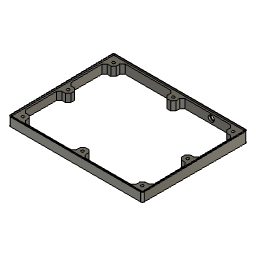
case (Autodesk Fusion 360 design; units mm, degrees)
Autodesk Fusion 360 part; units mm, degrees
sketch "Sketch1" plane through (0, 0, 0) normal (0, 0, 1) x (1, 0, 0)
  line L0 (0, 0) -> (294.692, 0)
  line L1 (294.692, 0) -> (294.692, 230.4)
  line L2 (294.692, 230.4) -> (0, 230.4)
  line L3 (0, 230.4) -> (0, 0)
  line L4 (-2, 232.4) -> (296.692, 232.4)
  line L5 (296.692, 232.4) -> (296.692, -2)
  line L6 (296.692, -2) -> (-2, -2)
  line L7 (-2, -2) -> (-2, 232.4)
  line L8 (4, 226.4) -> (290.692, 226.4)
  line L9 (290.692, 226.4) -> (290.692, 4)
  line L10 (290.692, 4) -> (4, 4)
  line L11 (4, 4) -> (4, 226.4)
  line L12 (4, 226.4) -> (24, 226.4)
  line L13 (24, 226.4) -> (24, 206.4)
  line L14 (24, 206.4) -> (4, 206.4)
  line L15 (4, 206.4) -> (4, 226.4)
  line L16 (-2, 232.4) -> (296.692, -2) construction
  line L17 (-2, -2) -> (296.692, 232.4) construction
  line L18 (-2, 115.2) -> (296.692, 115.2) construction
  line L19 (147.346, 232.4) -> (147.346, -2) construction
  line L20 (4, 206.4) -> (24, 226.4) construction
  line L21 (24, 206.4) -> (4, 226.4) construction
  line L22 (137.346, 226.4) -> (157.346, 226.4)
  line L23 (157.346, 226.4) -> (157.346, 206.4)
  line L24 (157.346, 206.4) -> (137.346, 206.4)
  line L25 (137.346, 206.4) -> (137.346, 226.4)
  line L26 (290.692, 226.4) -> (270.692, 226.4)
  line L27 (270.692, 226.4) -> (270.692, 206.4)
  line L28 (270.692, 206.4) -> (290.692, 206.4)
  line L29 (290.692, 206.4) -> (290.692, 226.4)
  line L30 (4, 125.2) -> (24, 125.2)
  line L31 (24, 125.2) -> (24, 105.2)
  line L32 (24, 105.2) -> (4, 105.2)
  line L33 (4, 105.2) -> (4, 125.2)
  line L34 (290.692, 125.2) -> (270.692, 125.2)
  line L35 (270.692, 125.2) -> (270.692, 105.2)
  line L36 (270.692, 105.2) -> (290.692, 105.2)
  line L37 (290.692, 105.2) -> (290.692, 125.2)
  line L38 (4, 4) -> (24, 4)
  line L39 (24, 4) -> (24, 24)
  line L40 (24, 24) -> (4, 24)
  line L41 (4, 24) -> (4, 4)
  line L42 (137.346, 4) -> (157.346, 4)
  line L43 (157.346, 4) -> (157.346, 24)
  line L44 (157.346, 24) -> (137.346, 24)
  line L45 (137.346, 24) -> (137.346, 4)
  line L46 (290.692, 4) -> (270.692, 4)
  line L47 (270.692, 4) -> (270.692, 24)
  line L48 (270.692, 24) -> (290.692, 24)
  line L49 (290.692, 24) -> (290.692, 4)
  line L50 (137.346, 206.4) -> (157.346, 226.4) construction
  line L51 (157.346, 206.4) -> (137.346, 226.4) construction
  line L52 (270.692, 206.4) -> (290.692, 226.4) construction
  line L53 (290.692, 206.4) -> (270.692, 226.4) construction
  line L54 (270.692, 105.2) -> (290.692, 125.2) construction
  line L55 (290.692, 105.2) -> (270.692, 125.2) construction
  line L56 (4, 105.2) -> (24, 125.2) construction
  line L57 (24, 105.2) -> (4, 125.2) construction
  line L58 (4, 4) -> (24, 24) construction
  line L59 (24, 4) -> (4, 24) construction
  line L60 (137.346, 4) -> (157.346, 24) construction
  line L61 (157.346, 4) -> (137.346, 24) construction
  line L62 (270.692, 4) -> (290.692, 24) construction
  line L63 (290.692, 4) -> (270.692, 24) construction
  circle A0 centre (14, 216.4) radius 3
  circle A1 centre (147.346, 216.4) radius 3
  circle A2 centre (280.692, 216.4) radius 3
  circle A3 centre (14, 115.2) radius 3
  circle A4 centre (280.692, 115.2) radius 3
  circle A5 centre (14, 14) radius 3
  circle A6 centre (147.346, 14) radius 3
  circle A7 centre (280.692, 14) radius 3
  dimension "d1" = 294.692
  dimension "d2" = 230.4
  dimension "d3" = 2
  dimension "d4" = 2
  dimension "d5" = 2
  dimension "d6" = 2
  dimension "d7" = 4
  dimension "d8" = 4
  dimension "d9" = 4
  dimension "d10" = 4
  dimension "d11" = 20
  dimension "d12" = 20
  dimension "d13" = 20
  dimension "d14" = 20
  dimension "d15" = 20
  dimension "d16" = 20
  dimension "d17" = 20
  dimension "d18" = 20
  dimension "d19" = 20
  dimension "d20" = 20
  dimension "d21" = 20
  dimension "d22" = 20
  dimension "d23" = 20
  dimension "d24" = 20
  dimension "d25" = 20
  dimension "d26" = 20
  dimension "d27" = 6
  dimension "d28" = 6
  dimension "d29" = 6
  dimension "d30" = 6
  dimension "d31" = 6
  dimension "d32" = 6
  dimension "d33" = 6
  dimension "d34" = 6
  constraint horizontal L0
  constraint vertical L1
  constraint horizontal L2
  constraint vertical L3
  constraint coincident L0.start L3.end
  constraint horizontal L4
  constraint vertical L5
  constraint horizontal L6
  constraint vertical L7
  constraint horizontal L8
  constraint vertical L9
  constraint horizontal L10
  constraint vertical L11
  constraint horizontal L12
  constraint vertical L13
  constraint horizontal L14
  constraint vertical L15
  constraint midpoint L7 L18.start
  constraint midpoint L5 L18.end
  constraint midpoint L4 L19.start
  constraint midpoint L6 L19.end
  constraint horizontal L22
  constraint vertical L23
  constraint horizontal L24
  constraint vertical L25
  constraint coincident L8 L22.start
  constraint horizontal L26
  constraint vertical L27
  constraint horizontal L28
  constraint vertical L29
  constraint horizontal L30
  constraint vertical L31
  constraint horizontal L32
  constraint vertical L33
  constraint coincident L11 L30.start
  constraint horizontal L34
  constraint vertical L35
  constraint horizontal L36
  constraint vertical L37
  constraint coincident L9 L34.start
  constraint horizontal L38
  constraint vertical L39
  constraint horizontal L40
  constraint vertical L41
  constraint horizontal L42
  constraint vertical L43
  constraint horizontal L44
  constraint vertical L45
  constraint coincident L10 L42.start
  constraint horizontal L46
  constraint vertical L47
  constraint horizontal L48
  constraint vertical L49
  constraint symmetric L19 L23 L25
  constraint symmetric L18 L30 L32
  constraint symmetric L18 L34 L36
  constraint symmetric L19 L43 L45
  constraint midpoint L21 A0.centre
  constraint midpoint L50 A1.centre
  constraint midpoint L53 A2.centre
  constraint midpoint L57 A3.centre
  constraint midpoint L54 A4.centre
  constraint midpoint L59 A5.centre
  constraint midpoint L60 A6.centre
  constraint midpoint L63 A7.centre
  measures "d1" distance of L0.start L0.end
  measures "d2" distance of L0.start L2.end
  measures "d3" distance of L2 L4
  measures "d4" distance of L3 L7
  measures "d5" distance of L0 L6
  measures "d6" distance of L1 L5
  measures "d7" distance of L3 L11
  measures "d8" distance of L0 L10
  measures "d9" distance of L2 L8
  measures "d10" distance of L1 L9
  measures "d11" distance of L8.start L12.end
  measures "d12" distance of L8.start L14.end
  measures "d13" distance of L22.start L22.end
  measures "d14" distance of L22.start L24.end
  measures "d15" distance of L8.end L26.end
  measures "d16" distance of L8.end L28.end
  measures "d17" distance of L30.start L30.end
  measures "d18" distance of L30.start L32.end
  measures "d19" distance of L34.start L34.end
  measures "d20" distance of L34.start L36.end
  measures "d21" distance of L10.end L38.end
  measures "d22" distance of L10.end L40.end
  measures "d23" distance of L42.start L42.end
  measures "d24" distance of L42.start L44.end
  measures "d25" distance of L9.end L46.end
  measures "d26" distance of L9.end L48.end
  measures "d27" diameter of A0
  measures "d28" diameter of A1
  measures "d29" diameter of A2
  measures "d30" diameter of A3
  measures "d31" diameter of A4
  measures "d32" diameter of A5
  measures "d33" diameter of A6
  measures "d34" diameter of A7
extrude "Extrude1" add sketch "Sketch1" along normal blind 20 contours L0 L1 L2 L3 | L4 L5 L6 L7 | L8 L11 L12 L13 L14 L15 | L8 L22 L23 L24 L25 | L11 L30 L31 L32 L33 | L8 L9 L26 L27 L28 L29 | L10 L11 L38 L39 L40 L41 | L9 L34 L35 L36 L37 | L10 L42 L43 L44 L45 | L9 L10 L46 L47 L48 L49
chamfer "Chamfer1" distance 6 angle 45 28 edges at (24, 206.4, 10) (4, 206.4, 10) (24, 226.4, 10) (137.346, 226.4, 10) (137.346, 206.4, 10) (157.346, 206.4, 10) (157.346, 226.4, 10) (270.692, 226.4, 10) (270.692, 206.4, 10) (290.692, 206.4, 10) (290.692, 125.2, 10) (270.692, 125.2, 10) (270.692, 105.2, 10) (290.692, 105.2, 10) (290.692, 24, 10) (270.692, 24, 10) (270.692, 4, 10) (157.346, 4, 10) (157.346, 24, 10) (137.346, 24, 10) (137.346, 4, 10) (24, 4, 10) (24, 24, 10) (4, 24, 10) (24, 105.2, 10) (4, 105.2, 10) (24, 125.2, 10) (4, 125.2, 10)
sketch "Sketch2" plane through (0, 0, 20) normal (0, 0, 1) x (-1, 0, 0)
  line L0 (-24, -119.2) -> (-18, -125.2)
  line L1 (-18, -125.2) -> (-10, -125.2)
  line L2 (-10, -125.2) -> (-4, -131.2)
  line L3 (-4, -131.2) -> (-4, -200.4)
  line L4 (-4, -200.4) -> (-10, -206.4)
  line L5 (-10, -206.4) -> (-18, -206.4)
  line L6 (-18, -206.4) -> (-24, -212.4)
  line L7 (-24, -212.4) -> (-24, -220.4)
  line L8 (-24, -220.4) -> (-30, -226.4)
  line L9 (-30, -226.4) -> (-131.346, -226.4)
  line L10 (-131.346, -226.4) -> (-137.346, -220.4)
  line L11 (-137.346, -220.4) -> (-137.346, -212.4)
  line L12 (-137.346, -212.4) -> (-143.346, -206.4)
  line L13 (-143.346, -206.4) -> (-151.346, -206.4)
  line L14 (-151.346, -206.4) -> (-157.346, -212.4)
  line L15 (-157.346, -212.4) -> (-157.346, -220.4)
  line L16 (-157.346, -220.4) -> (-163.346, -226.4)
  line L17 (-163.346, -226.4) -> (-264.692, -226.4)
  line L18 (-264.692, -226.4) -> (-270.692, -220.4)
  line L19 (-270.692, -220.4) -> (-270.692, -212.4)
  line L20 (-270.692, -212.4) -> (-276.692, -206.4)
  line L21 (-276.692, -206.4) -> (-284.692, -206.4)
  line L22 (-284.692, -206.4) -> (-290.692, -200.4)
  line L23 (-290.692, -200.4) -> (-290.692, -131.2)
  line L24 (-290.692, -131.2) -> (-284.692, -125.2)
  line L25 (-284.692, -125.2) -> (-276.692, -125.2)
  line L26 (-276.692, -125.2) -> (-270.692, -119.2)
  line L27 (-270.692, -119.2) -> (-270.692, -111.2)
  line L28 (-270.692, -111.2) -> (-276.692, -105.2)
  line L29 (-276.692, -105.2) -> (-284.692, -105.2)
  line L30 (-284.692, -105.2) -> (-290.692, -99.2)
  line L31 (-290.692, -99.2) -> (-290.692, -30)
  line L32 (-290.692, -30) -> (-284.692, -24)
  line L33 (-284.692, -24) -> (-276.692, -24)
  line L34 (-276.692, -24) -> (-270.692, -18)
  line L35 (-270.692, -18) -> (-270.692, -10)
  line L36 (-270.692, -10) -> (-264.692, -4)
  line L37 (-264.692, -4) -> (-163.346, -4)
  line L38 (-163.346, -4) -> (-157.346, -10)
  line L39 (-157.346, -10) -> (-157.346, -18)
  line L40 (-157.346, -18) -> (-151.346, -24)
  line L41 (-151.346, -24) -> (-143.346, -24)
  line L42 (-143.346, -24) -> (-137.346, -18)
  line L43 (-137.346, -18) -> (-137.346, -10)
  line L44 (-137.346, -10) -> (-131.346, -4)
  line L45 (-131.346, -4) -> (-30, -4)
  line L46 (-30, -4) -> (-24, -10)
  line L47 (-24, -10) -> (-24, -18)
  line L48 (-24, -18) -> (-18, -24)
  line L49 (-18, -24) -> (-10, -24)
  line L50 (-10, -24) -> (-4, -30)
  line L51 (-4, -30) -> (-4, -99.2)
  line L52 (-4, -99.2) -> (-10, -105.2)
  line L53 (-10, -105.2) -> (-18, -105.2)
  line L54 (-18, -105.2) -> (-24, -111.2)
  line L55 (-24, -111.2) -> (-24, -119.2)
  circle A0 centre (-280.692, -115.2) radius 3
  circle A1 centre (-280.692, -14) radius 3
  circle A2 centre (-147.346, -216.4) radius 3
  circle A3 centre (-14, -115.2) radius 3
  circle A4 centre (-14, -14) radius 3
  circle A5 centre (-280.692, -216.4) radius 3
  circle A6 centre (-147.346, -14) radius 3
  circle A7 centre (-14, -216.4) radius 3
  line L56 (2, 2) -> (-296.692, 2)
  line L57 (-296.692, 2) -> (-296.692, -232.4)
  line L58 (-296.692, -232.4) -> (2, -232.4)
  line L59 (2, -232.4) -> (2, 2)
  line L60 (0, -230.4) -> (-294.692, -230.4)
  line L61 (-294.692, -230.4) -> (-294.692, 0)
  line L62 (-294.692, 0) -> (0, 0)
  line L63 (0, 0) -> (0, -230.4)
  dimension "d38" = 2
  dimension "d39" = 2
  dimension "d40" = 2
  dimension "d41" = 2
  constraint horizontal L60
  constraint vertical L61
  constraint horizontal L62
  constraint vertical L63
  measures "d38" distance of L59 L63
  measures "d39" distance of L58 L60
  measures "d40" distance of L57 L61
  measures "d41" distance of L56 L62
sketch "Sketch3" plane through (-2, 0, 0) normal (-1, 0, 0) x (0, -1, 0)
  line L0 (-232.4, 0) -> (2, 0)
  line L1 (2, 0) -> (2, 20)
  line L2 (2, 20) -> (-232.4, 20)
  line L3 (-232.4, 20) -> (-232.4, 0)
  line L4 (2, 0) -> (2, 16)
  line L5 (2, 16) -> (-232.4, 20)
  dimension "d42" = 16
  constraint coincident L0.end L1.start
  constraint coincident L1 L4.end
  constraint coincident L2.end L3.start
  measures "d42" distance of L0.end L4.end
extrude "Extrude2" cut sketch "Sketch3" against normal through all contours L1 L2 L5
extrude "Extrude3" add sketch "Sketch2" against normal through all of body 1 contours L56 L57 L58 L59
extrude "Extrude4" add 1 faces at (196.4613, -1.3333, 20) along direction (0, 0, 1) blind 3
extrude "Extrude5" add sketch "Sketch1" against normal blind 2 contours L4 L5 L6 L7
sketch "Sketch4" plane through (-2, 0, 0) normal (-1, 0, 0) x (0, -1, 0)
  line L0 (-232.4, 23) -> (-232.4, -2)
  line L1 (-232.4, -2) -> (2, -2)
  line L2 (2, -2) -> (2, 23)
  line L3 (2, 23) -> (-232.4, 23)
  line L4 (2, -2) -> (2, 19)
  line L5 (2, 19) -> (-232.4, 23)
  dimension "d49" = 21
  constraint coincident L1.end L2.start
  constraint perpendicular L3 L4
  constraint coincident L0.start L3.end
  measures "d49" distance of L1.end L4.end
extrude "Extrude6" cut sketch "Sketch4" against normal through all contours L2 L3 L5
sketch "Sketch5" plane through (0, 232.4, 0) normal (0, 1, 0) x (-1, 0, 0)
  line L0 (2, -2) -> (2, 23)
  line L1 (2, 23) -> (-296.692, 23)
  line L2 (-296.692, 23) -> (-296.692, -2)
  line L3 (-296.692, -2) -> (2, -2)
  line L4 (-296.692, -2) -> (2, 23) construction
  line L5 (2, -2) -> (-296.692, 23) construction
  line L6 (-147.346, 23) -> (-147.346, -2) construction
  line L7 (-296.692, -2) -> (-147.346, 23) construction
  line L8 (-147.346, -2) -> (-296.692, 23) construction
  circle A0 centre (-222.019, 10.5) radius 6.3
  circle A1 centre (-222.019, 10.5) radius 6.8
  dimension "d51" = 12.6
  dimension "d52" = 13.6
  constraint coincident L2.end L3.start
  constraint coincident L0.end L1.start
  constraint coincident L0.start L3.end
  constraint coincident L1.end L2.start
  constraint midpoint L1 L6.start
  constraint midpoint L3 L6.end
  constraint midpoint L8 A0.centre
  constraint concentric A0 A1
  measures "d51" diameter of A0
  measures "d52" diameter of A1
extrude "Extrude7" cut sketch "Sketch5" against normal blind 6 contours A0 | A1
extrude "Extrude8" add sketch "Sketch5" against normal blind 2 contours A1
fillet "Fillet1" radius 4 4 edges at (296.692, 232.4, 10.5) (296.692, -2, 8.5) (-2, 232.4, 10.5) (-2, -2, 8.5)
fillet "Fillet2" radius 2 8 edges at (0, 230.4, 21.4659) (294.692, 230.4, 21.4659) (294.692, 0, 17.5341) (0, 0, 17.5341) (0, 0, -1) (294.692, 0, -1) (294.692, 230.4, -1) (0, 230.4, -1)
fillet "Fillet3" radius 1 16 edges at (-0.8284, 231.2284, 22.98) (-2, 115.2, 21) (-0.8284, -0.8284, 19.02) (147.346, -2, 19) (295.5204, -0.8284, 19.02) (296.692, 115.2, 21) (295.5204, 231.2284, 22.98) (147.346, 232.4, 23) (-0.8284, 231.2284, -2) (147.346, 232.4, -2) (295.5204, 231.2284, -2) (296.692, 115.2, -2) (295.5204, -0.8284, -2) (147.346, -2, -2) (-0.8284, -0.8284, -2) (-2, 115.2, -2)
equation "d49 = 16 mm + 2 mm + 3 mm"
